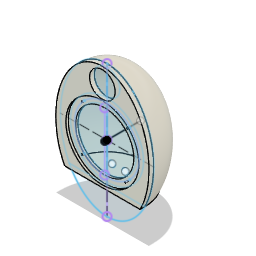
EggSpeak v8 (Autodesk Fusion 360 design; units mm, degrees)
Autodesk Fusion 360 part; units mm, degrees
sketch "Cone" plane through (0, 0, 0) normal (0, 0, 1) x (1, 0, 0)
  circle A0 centre (0, 65) radius 16.5
  circle A1 centre (29.2114, -29.4778) radius 1
  circle A2 centre (0, 0) radius 41.5
  circle A3 centre (0, 0) radius 47
  circle A4 centre (-29.2114, -29.4778) radius 1
  line L0 (-29.1972, 29.4919) -> (-29.1923, 29.4968)
  circle A5 centre (29.3721, 29.3319) radius 1
  circle A6 centre (0, 0) radius 37.5
  circle A7 centre (-29.1972, 29.4919) radius 1
sphere "SpherePrimitive1" add diameter 150 placed x (1, 0, 0) y (0, 1, 0) z (0, 0, 1) at (0, 10, 0) makes body 1
delete_face "DeleteFace1" 1 faces at (71.1056, 27.7286, -15.959) on bodies 1
sketch "Sketch4" plane through (0, 0, 0) normal (0, 0, 1) x (1, 0, 0)
  ellipse E0 centre (0, 0) end of major axis (0, 85.3485) minor radius 60
  line L0 (0, -85.3485) -> (0, 85.3485)
  line L1 (60, 0) -> (-60, 0)
  line L2 (-48.5705, -50.1088) -> (48.5705, -50.1088)
  line L3 (0, 85.3485) -> (0, -50.1088)
  constraint coincident E0.centre origin
  constraint vertical L0
  constraint coincident E0 L0.start
  constraint coincident E0 L0.end
  constraint coincident E0 L1.start
  constraint coincident E0 L1.end
  constraint coincident E0 L2.start
  constraint coincident E0 L2.end
  constraint horizontal L2
  constraint midpoint L2 L3.end
revolve "Revolve1" add sketch "Sketch4" angle 360 about axis through (0, 85.3485, 0) along (0, -1, 0) separate body contours E0 L0 L1 L3 | E0 L0 L1 L2 L3 picked at (39.6532, 5.2747) picked at (17.9382, -29.2836) makes body 2
extrude "Extrude2" cut sketch "Sketch4" along normal blind 60 contours E0 L0 L1 L3 | E0 L0 L1 L3 | E0 L0 L1 L2 L3 | E0 L0 L1 L2 L3 bodies 2
shell "Shell1" thickness 5 removed faces 1 at (-19.772, -9.9988, 0) on bodies 2
extrude "Extrude3" add sketch "Sketch4" along normal blind 6 separate body contours E0 L0 L1 L3 | E0 L0 L1 L3 | E0 L0 L1 L2 L3 | E0 L0 L1 L2 L3 makes body 3
extrude "Extrude4" cut sketch "Cone" along normal blind 35 contours A0 bodies 3
extrude "Extrude5" cut sketch "Cone" along normal blind 27 contours A6 bodies 3
extrude "Extrude6" cut sketch "Cone" along normal blind 8 and the other way blind -3 contours A1 A2 A4 A5 A7 | A3 bodies 3
extrude "Extrude7" cut 1 faces at (28.9007, 29.5343, 6) along direction (0, 0, -1) blind 12 on bodies 3 bodies 3
extrude "Extrude8" cut 1 faces at (-29.6686, 29.6944, 6) along direction (0, 0, -1) blind 15 on bodies 3 bodies 3
extrude "Extrude9" cut 1 faces at (-29.6966, -29.2148, 6) along direction (0, 0, -1) blind 31 on bodies 3 bodies 3
sketch "Sketch5" plane through (0, 0, 0) normal (1, 0, 0) x (0, 0, -1)
  line L0 (-3, 37.5) -> (-3, -37.5)
  line L1 (-3, 0) -> (43, 0)
  point P0 (-3, 0)
  constraint coincident P0 L1.start
  constraint perpendicular L0 L1
sketch "Binding Posts" plane through (0, 0, 0) normal (0, 0, 1) x (1, 0, 0)
  circle A0 through (11.9791, -38.1953, -15) (6.7291, -35.1642, -15) (6.7291, -41.2264, -15)
  circle A1 centre (0, 0) radius 41.5
  circle A2 through (-4.9791, -38.1953, -15) (-10.2291, -35.1642, -15) (-10.2291, -41.2264, -15)
  line L0 (0, -85.3485) -> (0, 85.3485)
extrude "Extrude10" [suppressed]
extrude "Extrude11" [suppressed]
extrude "Extrude12" [suppressed]
fillet "Fillet1" [suppressed]
combine "Combine1" [suppressed] in component "Component"
